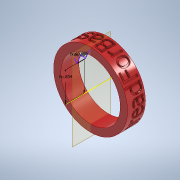
# Autodesk Inventor part: threadsForBaseV06
Saved by Autodesk Inventor 2021.1 (Build 251245010, 245A)
## iProperties
Created: 2020-08-18
Part Number: threadsForBaseV06
Material: PET Plastic
Document SubType Name: Modeling
Designer: robst
Density: 1.541 g/cm^3
Appearance: Red
Author: robst
Autodesk Inventor part; units mm, degrees
ref_plane "XZ Plane" through (0, 0, 0) normal (0, 1, 0) x (-1, 0, 0)
ref_plane "XY Plane" through (0, 0, 0) normal (0, 0, 1) x (1, 0, 0)
sketch "Sketch16" plane through (0, 0, 0) normal (0, 0, 1) x (1, 0, 0)
  circle A0 centre (0, 0) radius 21.1938
  circle A1 centre (0, 0) radius 26.3436
  dimension "d67" = 42.3875
  dimension "d68" = 52.6872
  constraints: 2 centre point, 2 coincident
  measures "d67" diameter of A0
  measures "d68" diameter of A1
extrude "Extrusion8" add sketch "Sketch16" against normal blind 12.7
ref_plane "Work Plane6" through (26.3436, 0, 0) normal (1, 0, 0) x (0, 1, 0)
sketch "Sketch18" plane through (26.3436, 0, 0) normal (1, 0, 0) x (0, 1, 0)
  line L0 (-26.3436, 0) -> (-26.3436, -12.7) projected
  line L1 (26.3436, 0) -> (26.3436, -12.7) projected
  line L2 (-26.3436, -6.35) -> (26.3436, -6.35) construction
  spline S0 degree 2 poles (-23.1079, -11.5782) (-24.1535, -11.5782) (-25.3309, -10.3844) (-25.3309, -9.0917) knots 0 0 0 1 2 2 2
  line L3 (-25.3309, -9.0917) -> (-25.3309, -4.868)
  line L4 (-25.3309, -4.868) -> (-26.1954, -4.868)
  line L5 (-26.1954, -4.868) -> (-26.1954, -3.8059)
  line L6 (-26.1954, -3.8059) -> (-25.3309, -3.8059)
  line L7 (-25.3309, -3.8059) -> (-25.3309, -1.6158)
  line L8 (-25.3309, -1.6158) -> (-24.0465, -1.6158)
  line L9 (-24.0465, -1.6158) -> (-24.0465, -3.8059)
  line L10 (-24.0465, -3.8059) -> (-21.6835, -3.8059)
  line L11 (-21.6835, -3.8059) -> (-21.6835, -4.868)
  line L12 (-21.6835, -4.868) -> (-24.0465, -4.868)
  line L13 (-24.0465, -4.868) -> (-24.0465, -8.4989)
  spline S1 degree 2 poles (-24.0465, -8.4989) (-24.0465, -9.0753) (-24.0053, -9.7092) (-23.8654, -9.9809) knots 0 0 0 1 2 2 2
  spline S2 degree 2 poles (-23.8654, -9.9809) (-23.7501, -10.2197) (-23.2314, -10.4585) (-22.7868, -10.4585) knots 0 0 0 1 2 2 2
  spline S3 degree 2 poles (-22.7868, -10.4585) (-22.4739, -10.4585) (-21.8893, -10.2691) (-21.7576, -10.2115) knots 0 0 0 1 2 2 2
  line L14 (-21.7576, -10.2115) -> (-21.6835, -10.2115)
  line L15 (-21.6835, -10.2115) -> (-21.6835, -11.3641)
  spline S4 degree 2 poles (-21.6835, -11.3641) (-22.0458, -11.4629) (-22.7868, -11.5782) (-23.1079, -11.5782) knots 0 0 0 1 2 2 2
  line L16 (-14.751, -11.43) -> (-16.0354, -11.43)
  line L17 (-16.0354, -11.43) -> (-16.0354, -7.0828)
  spline S5 degree 2 poles (-16.0354, -7.0828) (-16.0354, -6.5558) (-16.1342, -5.6502) (-16.2824, -5.3785) knots 0 0 0 1 2 2 2
  spline S6 degree 2 poles (-16.2824, -5.3785) (-16.4388, -5.0903) (-16.9987, -4.8104) (-17.4763, -4.8104) knots 0 0 0 1 2 2 2
  spline S7 degree 2 poles (-17.4763, -4.8104) (-17.9538, -4.8104) (-18.9665, -5.3208) (-19.4523, -5.7325) knots 0 0 0 1 2 2 2
  line L18 (-19.4523, -5.7325) -> (-19.4523, -11.43)
  line L19 (-19.4523, -11.43) -> (-20.7367, -11.43)
  line L20 (-20.7367, -11.43) -> (-20.7367, -0.8172)
  line L21 (-20.7367, -0.8172) -> (-19.4523, -0.8172)
  line L22 (-19.4523, -0.8172) -> (-19.4523, -4.6539)
  spline S8 degree 2 poles (-19.4523, -4.6539) (-18.8759, -4.1352) (-17.7644, -3.5918) (-17.1387, -3.5918) knots 0 0 0 1 2 2 2
  spline S9 degree 2 poles (-17.1387, -3.5918) (-16.0189, -3.5918) (-14.751, -5.0738) (-14.751, -6.4817) knots 0 0 0 1 2 2 2
  line L23 (-14.751, -6.4817) -> (-14.751, -11.43)
  line L24 (-8.9053, -5.1809) -> (-8.9712, -5.1809)
  spline S10 degree 2 poles (-8.9712, -5.1809) (-9.1194, -5.1397) (-9.4405, -5.1232) (-9.6628, -5.1232) knots 0 0 0 1 2 2 2
  spline S11 degree 2 poles (-9.6628, -5.1232) (-10.1815, -5.1232) (-11.2024, -5.5761) (-11.6635, -6.0207) knots 0 0 0 1 2 2 2
  line L25 (-11.6635, -6.0207) -> (-11.6635, -11.43)
  line L26 (-11.6635, -11.43) -> (-12.9479, -11.43)
  line L27 (-12.9479, -11.43) -> (-12.9479, -3.8059)
  line L28 (-12.9479, -3.8059) -> (-11.6635, -3.8059)
  line L29 (-11.6635, -3.8059) -> (-11.6635, -4.9421)
  spline S12 degree 2 poles (-11.6635, -4.9421) (-10.9636, -4.3164) (-9.918, -3.8059) (-9.424, -3.8059) knots 0 0 0 1 2 2 2
  spline S13 degree 2 poles (-9.424, -3.8059) (-9.2264, -3.8059) (-9.0288, -3.8223) (-8.9053, -3.8471) knots 0 0 0 1 2 2 2
  line L30 (-8.9053, -3.8471) -> (-8.9053, -5.1809)
  spline S14 degree 2 poles (-4.5992, -11.6029) (-6.427, -11.6029) (-8.436, -9.5528) (-8.436, -7.6591) knots 0 0 0 1 2 2 2
  spline S15 degree 2 poles (-8.436, -7.6591) (-8.436, -5.7984) (-6.4847, -3.5918) (-4.9121, -3.5918) knots 0 0 0 1 2 2 2
  spline S16 degree 2 poles (-4.9121, -3.5918) (-4.204, -3.5918) (-3.109, -4.0035) (-2.7056, -4.4399) knots 0 0 0 1 2 2 2
  spline S17 degree 2 poles (-2.7056, -4.4399) (-2.2939, -4.8762) (-1.8575, -6.1359) (-1.8575, -7.0498) knots 0 0 0 1 2 2 2
  line L31 (-1.8575, -7.0498) -> (-1.8575, -7.7497)
  line L32 (-1.8575, -7.7497) -> (-7.1351, -7.7497)
  spline S18 degree 2 poles (-7.1351, -7.7497) (-7.1351, -9.0753) (-5.8013, -10.4832) (-4.6157, -10.4832) knots 0 0 0 1 2 2 2
  spline S19 degree 2 poles (-4.6157, -10.4832) (-4.1958, -10.4832) (-3.3807, -10.2938) (-3.0514, -10.1456) knots 0 0 0 1 2 2 2
  spline S20 degree 2 poles (-3.0514, -10.1456) (-2.7056, -9.9809) (-2.228, -9.6928) (-2.0716, -9.561) knots 0 0 0 1 2 2 2
  line L33 (-2.0716, -9.561) -> (-1.9975, -9.561)
  line L34 (-1.9975, -9.561) -> (-1.9975, -10.9607)
  spline S21 degree 2 poles (-1.9975, -10.9607) (-2.2198, -11.0513) (-2.8949, -11.3147) (-3.1584, -11.3888) knots 0 0 0 1 2 2 2
  spline S22 degree 2 poles (-3.1584, -11.3888) (-3.5289, -11.4959) (-4.1382, -11.6029) (-4.5992, -11.6029) knots 0 0 0 1 2 2 2
  spline S23 degree 2 poles (-3.109, -6.7699) (-3.1255, -6.2512) (-3.3395, -5.4937) (-3.5454, -5.2385) knots 0 0 0 1 2 2 2
  spline S24 degree 2 poles (-3.5454, -5.2385) (-3.7677, -4.9503) (-4.4675, -4.6457) (-4.9862, -4.6457) knots 0 0 0 1 2 2 2
  spline S25 degree 2 poles (-4.9862, -4.6457) (-5.4967, -4.6457) (-6.213, -4.9503) (-6.5094, -5.2467) knots 0 0 0 1 2 2 2
  spline S26 degree 2 poles (-6.5094, -5.2467) (-6.7975, -5.5514) (-7.094, -6.2841) (-7.1351, -6.7699) knots 0 0 0 1 2 2 2
  line L35 (-7.1351, -6.7699) -> (-3.109, -6.7699)
  spline S27 degree 2 poles (3.6918, -10.6231) (3.5354, -10.7384) (3.0084, -11.1501) (2.7614, -11.2736) knots 0 0 0 1 2 2 2
  spline S28 degree 2 poles (2.7614, -11.2736) (2.4238, -11.4547) (1.7899, -11.6441) (1.2135, -11.6441) knots 0 0 0 1 2 2 2
  spline S29 degree 2 poles (1.2135, -11.6441) (0.7442, -11.6441) (-0.1038, -11.29) (-0.4249, -10.9689) knots 0 0 0 1 2 2 2
  spline S30 degree 2 poles (-0.4249, -10.9689) (-0.7295, -10.6561) (-1.1, -9.7339) (-1.1, -9.2235) knots 0 0 0 1 2 2 2
  spline S31 degree 2 poles (-1.1, -9.2235) (-1.1, -8.433) (-0.4331, -7.3133) (0.2914, -6.9922) knots 0 0 0 1 2 2 2
  spline S32 degree 2 poles (0.2914, -6.9922) (0.9336, -6.6958) (2.6791, -6.4735) (3.6918, -6.4159) knots 0 0 0 1 2 2 2
  line L36 (3.6918, -6.4159) -> (3.6918, -6.1689)
  spline S33 degree 2 poles (3.6918, -6.1689) (3.6918, -5.7243) (3.4201, -5.1726) (3.1731, -5.0162) knots 0 0 0 1 2 2 2
  spline S34 degree 2 poles (3.1731, -5.0162) (2.9261, -4.8598) (2.218, -4.761) (1.8393, -4.761) knots 0 0 0 1 2 2 2
  spline S35 degree 2 poles (1.8393, -4.761) (1.3947, -4.761) (0.1926, -5.0244) (-0.4084, -5.2797) knots 0 0 0 1 2 2 2
  line L37 (-0.4084, -5.2797) -> (-0.4825, -5.2797)
  line L38 (-0.4825, -5.2797) -> (-0.4825, -3.9706)
  spline S36 degree 2 poles (-0.4825, -3.9706) (-0.1285, -3.8718) (1.1971, -3.6247) (1.8475, -3.6247) knots 0 0 0 1 2 2 2
  spline S37 degree 2 poles (1.8475, -3.6247) (2.6379, -3.6247) (3.7165, -3.8718) (4.1446, -4.1929) knots 0 0 0 1 2 2 2
  spline S38 degree 2 poles (4.1446, -4.1929) (4.5645, -4.5057) (4.9762, -5.502) (4.9762, -6.2183) knots 0 0 0 1 2 2 2
  line L39 (4.9762, -6.2183) -> (4.9762, -11.43)
  line L40 (4.9762, -11.43) -> (3.6918, -11.43)
  line L41 (3.6918, -11.43) -> (3.6918, -10.6231)
  line L42 (3.6918, -9.5528) -> (3.6918, -7.4368)
  spline S39 degree 2 poles (3.6918, -7.4368) (3.2307, -7.478) (1.8393, -7.6179) (1.4029, -7.7497) knots 0 0 0 1 2 2 2
  spline S40 degree 2 poles (1.4029, -7.7497) (0.8924, -7.9061) (0.2255, -8.5565) (0.2255, -9.1329) knots 0 0 0 1 2 2 2
  spline S41 degree 2 poles (0.2255, -9.1329) (0.2255, -9.7916) (0.9665, -10.4585) (1.6746, -10.4585) knots 0 0 0 1 2 2 2
  spline S42 degree 2 poles (1.6746, -10.4585) (2.2756, -10.4585) (3.2637, -9.9398) (3.6918, -9.5528) knots 0 0 0 1 2 2 2
  line L43 (12.6415, -11.43) -> (11.3571, -11.43)
  line L44 (11.3571, -11.43) -> (11.3571, -10.6561)
  spline S43 degree 2 poles (11.3571, -10.6561) (11.0607, -10.9031) (10.6243, -11.2324) (10.3279, -11.3724) knots 0 0 0 1 2 2 2
  spline S44 degree 2 poles (10.3279, -11.3724) (10.0562, -11.5041) (9.4716, -11.6441) (9.0847, -11.6441) knots 0 0 0 1 2 2 2
  spline S45 degree 2 poles (9.0847, -11.6441) (8.4589, -11.6441) (7.405, -11.1254) (7.0345, -10.6231) knots 0 0 0 1 2 2 2
  spline S46 degree 2 poles (7.0345, -10.6231) (6.664, -10.1209) (6.2524, -8.6389) (6.2524, -7.6756) knots 0 0 0 1 2 2 2
  spline S47 degree 2 poles (6.2524, -7.6756) (6.2524, -6.6711) (6.7711, -5.2056) (7.2239, -4.6539) knots 0 0 0 1 2 2 2
  spline S48 degree 2 poles (7.2239, -4.6539) (7.6438, -4.1599) (8.8212, -3.5918) (9.4716, -3.5918) knots 0 0 0 1 2 2 2
  spline S49 degree 2 poles (9.4716, -3.5918) (10.0397, -3.5918) (10.8878, -3.8471) (11.3571, -4.1105) knots 0 0 0 1 2 2 2
  line L45 (11.3571, -4.1105) -> (11.3571, -0.8172)
  line L46 (11.3571, -0.8172) -> (12.6415, -0.8172)
  line L47 (12.6415, -0.8172) -> (12.6415, -11.43)
  line L48 (11.3571, -9.5775) -> (11.3571, -5.1726)
  spline S50 degree 2 poles (11.3571, -5.1726) (10.8795, -4.9421) (10.1221, -4.7692) (9.6857, -4.7692) knots 0 0 0 1 2 2 2
  spline S51 degree 2 poles (9.6857, -4.7692) (8.6977, -4.7692) (7.5779, -6.2512) (7.5779, -7.6509) knots 0 0 0 1 2 2 2
  spline S52 degree 2 poles (7.5779, -7.6509) (7.5779, -9.0012) (8.4342, -10.4255) (9.3811, -10.4255) knots 0 0 0 1 2 2 2
  spline S53 degree 2 poles (9.3811, -10.4255) (9.8833, -10.4255) (10.9042, -9.9645) (11.3571, -9.5775) knots 0 0 0 1 2 2 2
  line L49 (20.6773, -2.4721) -> (15.9513, -2.4721)
  line L50 (15.9513, -2.4721) -> (15.9513, -5.3373)
  line L51 (15.9513, -5.3373) -> (20.4797, -5.3373)
  line L52 (20.4797, -5.3373) -> (20.4797, -6.5394)
  line L53 (20.4797, -6.5394) -> (15.9513, -6.5394)
  line L54 (15.9513, -6.5394) -> (15.9513, -11.43)
  line L55 (15.9513, -11.43) -> (14.601, -11.43)
  line L56 (14.601, -11.43) -> (14.601, -1.27)
  line L57 (14.601, -1.27) -> (20.6773, -1.27)
  line L58 (20.6773, -1.27) -> (20.6773, -2.4721)
  spline S54 degree 2 poles (28.0544, -7.6179) (28.0544, -9.5446) (26.2019, -11.6441) (24.654, -11.6441) knots 0 0 0 1 2 2 2
  spline S55 degree 2 poles (24.654, -11.6441) (23.0649, -11.6441) (21.2454, -9.4787) (21.2454, -7.6179) knots 0 0 0 1 2 2 2
  spline S56 degree 2 poles (21.2454, -7.6179) (21.2454, -5.7078) (23.1226, -3.5918) (24.654, -3.5918) knots 0 0 0 1 2 2 2
  spline S57 degree 2 poles (24.654, -3.5918) (26.2019, -3.5918) (28.0544, -5.6996) (28.0544, -7.6179) knots 0 0 0 1 2 2 2
  spline S58 degree 2 poles (26.7288, -7.6179) (26.7288, -6.1359) (25.6502, -4.6951) (24.654, -4.6951) knots 0 0 0 1 2 2 2
  spline S59 degree 2 poles (24.654, -4.6951) (23.6578, -4.6951) (22.5709, -6.1359) (22.5709, -7.6179) knots 0 0 0 1 2 2 2
  spline S60 degree 2 poles (22.5709, -7.6179) (22.5709, -9.0588) (23.6578, -10.5408) (24.654, -10.5408) knots 0 0 0 1 2 2 2
  spline S61 degree 2 poles (24.654, -10.5408) (25.642, -10.5408) (26.7288, -9.0835) (26.7288, -7.6179) knots 0 0 0 1 2 2 2
  line L59 (33.4143, -5.1809) -> (33.3484, -5.1809)
  spline S62 degree 2 poles (33.3484, -5.1809) (33.2002, -5.1397) (32.8791, -5.1232) (32.6568, -5.1232) knots 0 0 0 1 2 2 2
  spline S63 degree 2 poles (32.6568, -5.1232) (32.1381, -5.1232) (31.1172, -5.5761) (30.6561, -6.0207) knots 0 0 0 1 2 2 2
  line L60 (30.6561, -6.0207) -> (30.6561, -11.43)
  line L61 (30.6561, -11.43) -> (29.3717, -11.43)
  line L62 (29.3717, -11.43) -> (29.3717, -3.8059)
  line L63 (29.3717, -3.8059) -> (30.6561, -3.8059)
  line L64 (30.6561, -3.8059) -> (30.6561, -4.9421)
  spline S64 degree 2 poles (30.6561, -4.9421) (31.356, -4.3164) (32.4016, -3.8059) (32.8956, -3.8059) knots 0 0 0 1 2 2 2
  spline S65 degree 2 poles (32.8956, -3.8059) (33.0932, -3.8059) (33.2908, -3.8223) (33.4143, -3.8471) knots 0 0 0 1 2 2 2
  line L65 (33.4143, -3.8471) -> (33.4143, -5.1809)
  spline S66 degree 2 poles (41.4007, -8.3095) (41.4007, -9.067) (40.8244, -10.2279) (40.3468, -10.6067) knots 0 0 0 1 2 2 2
  spline S67 degree 2 poles (40.3468, -10.6067) (39.7705, -11.0513) (38.4614, -11.43) (37.424, -11.43) knots 0 0 0 1 2 2 2
  line L66 (37.424, -11.43) -> (34.5094, -11.43)
  line L67 (34.5094, -11.43) -> (34.5094, -1.27)
  line L68 (34.5094, -1.27) -> (37.2017, -1.27)
  spline S68 degree 2 poles (37.2017, -1.27) (38.2885, -1.27) (39.3753, -1.41) (39.8693, -1.6817) knots 0 0 0 1 2 2 2
  spline S69 degree 2 poles (39.8693, -1.6817) (40.4209, -1.9698) (40.9232, -2.9167) (40.9232, -3.5589) knots 0 0 0 1 2 2 2
  spline S70 degree 2 poles (40.9232, -3.5589) (40.9232, -4.2752) (40.1657, -5.4114) (39.4988, -5.7325) knots 0 0 0 1 2 2 2
  line L69 (39.4988, -5.7325) -> (39.4988, -5.7819)
  spline S71 degree 2 poles (39.4988, -5.7819) (40.4045, -6.0289) (41.4007, -7.338) (41.4007, -8.3095) knots 0 0 0 1 2 2 2
  spline S72 degree 2 poles (39.9928, -8.3672) (39.9928, -7.7908) (39.6635, -7.0498) (39.1695, -6.7864) knots 0 0 0 1 2 2 2
  spline S73 degree 2 poles (39.1695, -6.7864) (38.8484, -6.6217) (38.0909, -6.5229) (37.391, -6.5229) knots 0 0 0 1 2 2 2
  line L70 (37.391, -6.5229) -> (35.8596, -6.5229)
  line L71 (35.8596, -6.5229) -> (35.8596, -10.2773)
  line L72 (35.8596, -10.2773) -> (36.9547, -10.2773)
  spline S74 degree 2 poles (36.9547, -10.2773) (37.8439, -10.2773) (38.8648, -10.1127) (39.26, -9.8492) knots 0 0 0 1 2 2 2
  spline S75 degree 2 poles (39.26, -9.8492) (39.6388, -9.5775) (39.9928, -8.9024) (39.9928, -8.3672) knots 0 0 0 1 2 2 2
  spline S76 degree 2 poles (39.5153, -3.7482) (39.5153, -3.386) (39.2683, -2.8426) (38.9966, -2.6861) knots 0 0 0 1 2 2 2
  spline S77 degree 2 poles (38.9966, -2.6861) (38.6672, -2.505) (37.8686, -2.4227) (37.1523, -2.4227) knots 0 0 0 1 2 2 2
  line L73 (37.1523, -2.4227) -> (35.8596, -2.4227)
  line L74 (35.8596, -2.4227) -> (35.8596, -5.3949)
  line L75 (35.8596, -5.3949) -> (37.391, -5.3949)
  spline S78 degree 2 poles (37.391, -5.3949) (38.025, -5.3949) (38.6261, -5.2632) (38.9472, -5.0574) knots 0 0 0 1 2 2 2
  spline S79 degree 2 poles (38.9472, -5.0574) (39.26, -4.8598) (39.5153, -4.2258) (39.5153, -3.7482) knots 0 0 0 1 2 2 2
  spline S80 degree 2 poles (46.8924, -10.6231) (46.7359, -10.7384) (46.209, -11.1501) (45.962, -11.2736) knots 0 0 0 1 2 2 2
  spline S81 degree 2 poles (45.962, -11.2736) (45.6244, -11.4547) (44.9905, -11.6441) (44.4141, -11.6441) knots 0 0 0 1 2 2 2
  spline S82 degree 2 poles (44.4141, -11.6441) (43.9448, -11.6441) (43.0968, -11.29) (42.7757, -10.9689) knots 0 0 0 1 2 2 2
  spline S83 degree 2 poles (42.7757, -10.9689) (42.471, -10.6561) (42.1005, -9.7339) (42.1005, -9.2235) knots 0 0 0 1 2 2 2
  spline S84 degree 2 poles (42.1005, -9.2235) (42.1005, -8.433) (42.7674, -7.3133) (43.492, -6.9922) knots 0 0 0 1 2 2 2
  spline S85 degree 2 poles (43.492, -6.9922) (44.1342, -6.6958) (45.8797, -6.4735) (46.8924, -6.4159) knots 0 0 0 1 2 2 2
  line L76 (46.8924, -6.4159) -> (46.8924, -6.1689)
  spline S86 degree 2 poles (46.8924, -6.1689) (46.8924, -5.7243) (46.6207, -5.1726) (46.3737, -5.0162) knots 0 0 0 1 2 2 2
  spline S87 degree 2 poles (46.3737, -5.0162) (46.1267, -4.8598) (45.4186, -4.761) (45.0399, -4.761) knots 0 0 0 1 2 2 2
  spline S88 degree 2 poles (45.0399, -4.761) (44.5953, -4.761) (43.3932, -5.0244) (42.7921, -5.2797) knots 0 0 0 1 2 2 2
  line L77 (42.7921, -5.2797) -> (42.718, -5.2797)
  line L78 (42.718, -5.2797) -> (42.718, -3.9706)
  spline S89 degree 2 poles (42.718, -3.9706) (43.0721, -3.8718) (44.3977, -3.6247) (45.0481, -3.6247) knots 0 0 0 1 2 2 2
  spline S90 degree 2 poles (45.0481, -3.6247) (45.8385, -3.6247) (46.9171, -3.8718) (47.3452, -4.1929) knots 0 0 0 1 2 2 2
  spline S91 degree 2 poles (47.3452, -4.1929) (47.7651, -4.5057) (48.1768, -5.502) (48.1768, -6.2183) knots 0 0 0 1 2 2 2
  line L79 (48.1768, -6.2183) -> (48.1768, -11.43)
  line L80 (48.1768, -11.43) -> (46.8924, -11.43)
  line L81 (46.8924, -11.43) -> (46.8924, -10.6231)
  line L82 (46.8924, -9.5528) -> (46.8924, -7.4368)
  spline S92 degree 2 poles (46.8924, -7.4368) (46.4313, -7.478) (45.0399, -7.6179) (44.6035, -7.7497) knots 0 0 0 1 2 2 2
  spline S93 degree 2 poles (44.6035, -7.7497) (44.093, -7.9061) (43.4261, -8.5565) (43.4261, -9.1329) knots 0 0 0 1 2 2 2
  spline S94 degree 2 poles (43.4261, -9.1329) (43.4261, -9.7916) (44.1671, -10.4585) (44.8752, -10.4585) knots 0 0 0 1 2 2 2
  spline S95 degree 2 poles (44.8752, -10.4585) (45.4762, -10.4585) (46.4642, -9.9398) (46.8924, -9.5528) knots 0 0 0 1 2 2 2
  spline S96 degree 2 poles (52.0382, -11.6111) (51.2725, -11.6111) (49.947, -11.1995) (49.5106, -10.9689) knots 0 0 0 1 2 2 2
  line L83 (49.5106, -10.9689) -> (49.5106, -9.5281)
  line L84 (49.5106, -9.5281) -> (49.5765, -9.5281)
  spline S97 degree 2 poles (49.5765, -9.5281) (49.7411, -9.6598) (50.1857, -9.9727) (50.5562, -10.1456) knots 0 0 0 1 2 2 2
  spline S98 degree 2 poles (50.5562, -10.1456) (50.8773, -10.302) (51.6677, -10.5326) (52.0876, -10.5326) knots 0 0 0 1 2 2 2
  spline S99 degree 2 poles (52.0876, -10.5326) (52.3923, -10.5326) (53.0921, -10.3926) (53.2568, -10.2773) knots 0 0 0 1 2 2 2
  spline S100 degree 2 poles (53.2568, -10.2773) (53.4955, -10.1209) (53.7096, -9.7669) (53.7096, -9.4046) knots 0 0 0 1 2 2 2
  spline S101 degree 2 poles (53.7096, -9.4046) (53.7096, -8.9518) (53.2156, -8.4824) (52.5816, -8.326) knots 0 0 0 1 2 2 2
  spline S102 degree 2 poles (52.5816, -8.326) (52.3346, -8.2684) (51.5442, -8.1037) (51.2067, -8.0131) knots 0 0 0 1 2 2 2
  spline S103 degree 2 poles (51.2067, -8.0131) (50.3339, -7.7579) (49.5435, -6.704) (49.5435, -5.9548) knots 0 0 0 1 2 2 2
  spline S104 degree 2 poles (49.5435, -5.9548) (49.5435, -4.9174) (51.0996, -3.6247) (52.384, -3.6247) knots 0 0 0 1 2 2 2
  spline S105 degree 2 poles (52.384, -3.6247) (53.018, -3.6247) (54.3024, -3.9376) (54.7388, -4.1764) knots 0 0 0 1 2 2 2
  line L85 (54.7388, -4.1764) -> (54.7388, -5.5514)
  line L86 (54.7388, -5.5514) -> (54.6729, -5.5514)
  spline S106 degree 2 poles (54.6729, -5.5514) (54.1789, -5.1562) (52.9768, -4.7033) (52.3593, -4.7033) knots 0 0 0 1 2 2 2
  spline S107 degree 2 poles (52.3593, -4.7033) (51.7254, -4.7033) (50.8526, -5.2385) (50.8526, -5.7737) knots 0 0 0 1 2 2 2
  spline S108 degree 2 poles (50.8526, -5.7737) (50.8526, -6.2594) (51.3713, -6.7287) (51.9477, -6.8769) knots 0 0 0 1 2 2 2
  spline S109 degree 2 poles (51.9477, -6.8769) (52.2276, -6.951) (52.9357, -7.0992) (53.3226, -7.1898) knots 0 0 0 1 2 2 2
  spline S110 degree 2 poles (53.3226, -7.1898) (54.1625, -7.4039) (55.0187, -8.3836) (55.0187, -9.2317) knots 0 0 0 1 2 2 2
  spline S111 degree 2 poles (55.0187, -9.2317) (55.0187, -9.7257) (54.6318, -10.5984) (54.253, -10.9195) knots 0 0 0 1 2 2 2
  spline S112 degree 2 poles (54.253, -10.9195) (53.8496, -11.2571) (52.8204, -11.6111) (52.0382, -11.6111) knots 0 0 0 1 2 2 2
  spline S113 degree 2 poles (59.5224, -11.6029) (57.6946, -11.6029) (55.6856, -9.5528) (55.6856, -7.6591) knots 0 0 0 1 2 2 2
  spline S114 degree 2 poles (55.6856, -7.6591) (55.6856, -5.7984) (57.6369, -3.5918) (59.2095, -3.5918) knots 0 0 0 1 2 2 2
  spline S115 degree 2 poles (59.2095, -3.5918) (59.9176, -3.5918) (61.0126, -4.0035) (61.4161, -4.4399) knots 0 0 0 1 2 2 2
  spline S116 degree 2 poles (61.4161, -4.4399) (61.8277, -4.8762) (62.2641, -6.1359) (62.2641, -7.0498) knots 0 0 0 1 2 2 2
  line L87 (62.2641, -7.0498) -> (62.2641, -7.7497)
  line L88 (62.2641, -7.7497) -> (56.9865, -7.7497)
  spline S117 degree 2 poles (56.9865, -7.7497) (56.9865, -9.0753) (58.3203, -10.4832) (59.5059, -10.4832) knots 0 0 0 1 2 2 2
  spline S118 degree 2 poles (59.5059, -10.4832) (59.9258, -10.4832) (60.7409, -10.2938) (61.0703, -10.1456) knots 0 0 0 1 2 2 2
  spline S119 degree 2 poles (61.0703, -10.1456) (61.4161, -9.9809) (61.8936, -9.6928) (62.05, -9.561) knots 0 0 0 1 2 2 2
  line L89 (62.05, -9.561) -> (62.1241, -9.561)
  line L90 (62.1241, -9.561) -> (62.1241, -10.9607)
  spline S120 degree 2 poles (62.1241, -10.9607) (61.9018, -11.0513) (61.2267, -11.3147) (60.9632, -11.3888) knots 0 0 0 1 2 2 2
  spline S121 degree 2 poles (60.9632, -11.3888) (60.5927, -11.4959) (59.9835, -11.6029) (59.5224, -11.6029) knots 0 0 0 1 2 2 2
  spline S122 degree 2 poles (61.0126, -6.7699) (60.9962, -6.2512) (60.7821, -5.4937) (60.5763, -5.2385) knots 0 0 0 1 2 2 2
  spline S123 degree 2 poles (60.5763, -5.2385) (60.354, -4.9503) (59.6541, -4.6457) (59.1354, -4.6457) knots 0 0 0 1 2 2 2
  spline S124 degree 2 poles (59.1354, -4.6457) (58.6249, -4.6457) (57.9086, -4.9503) (57.6122, -5.2467) knots 0 0 0 1 2 2 2
  spline S125 degree 2 poles (57.6122, -5.2467) (57.3241, -5.5514) (57.0277, -6.2841) (56.9865, -6.7699) knots 0 0 0 1 2 2 2
  line L91 (56.9865, -6.7699) -> (61.0126, -6.7699)
  line L92 (75.3964, -1.27) -> (71.8972, -11.43)
  line L93 (71.8972, -11.43) -> (70.4399, -11.43)
  line L94 (70.4399, -11.43) -> (66.9407, -1.27)
  line L95 (66.9407, -1.27) -> (68.3897, -1.27)
  line L96 (68.3897, -1.27) -> (71.2056, -9.7092)
  line L97 (71.2056, -9.7092) -> (74.0214, -1.27)
  line L98 (74.0214, -1.27) -> (75.3964, -1.27)
  spline S126 degree 2 poles (82.5182, -6.35) (82.5182, -9.0835) (80.9292, -11.6441) (79.2743, -11.6441) knots 0 0 0 1 2 2 2
  spline S127 degree 2 poles (79.2743, -11.6441) (77.5947, -11.6441) (76.0221, -9.0341) (76.0221, -6.3582) knots 0 0 0 1 2 2 2
  spline S128 degree 2 poles (76.0221, -6.3582) (76.0221, -3.6083) (77.6111, -1.0642) (79.2743, -1.0642) knots 0 0 0 1 2 2 2
  spline S129 degree 2 poles (79.2743, -1.0642) (80.9457, -1.0642) (82.5182, -3.6988) (82.5182, -6.35) knots 0 0 0 1 2 2 2
  spline S130 degree 2 poles (80.7728, -9.4458) (80.9704, -8.9435) (81.135, -7.3956) (81.135, -6.35) knots 0 0 0 1 2 2 2
  spline S131 degree 2 poles (81.135, -6.35) (81.135, -5.3044) (80.9704, -3.7647) (80.7645, -3.246) knots 0 0 0 1 2 2 2
  spline S132 degree 2 poles (80.7645, -3.246) (80.5587, -2.7273) (79.8424, -2.1921) (79.2743, -2.1921) knots 0 0 0 1 2 2 2
  spline S133 degree 2 poles (79.2743, -2.1921) (78.7062, -2.1921) (77.9734, -2.7273) (77.7593, -3.2625) knots 0 0 0 1 2 2 2
  spline S134 degree 2 poles (77.7593, -3.2625) (77.5535, -3.7812) (77.4053, -5.362) (77.4053, -6.3582) knots 0 0 0 1 2 2 2
  spline S135 degree 2 poles (77.4053, -6.3582) (77.4053, -7.4286) (77.537, -8.8612) (77.7511, -9.4211) knots 0 0 0 1 2 2 2
  spline S136 degree 2 poles (77.7511, -9.4211) (77.9487, -9.948) (78.6815, -10.5161) (79.2743, -10.5161) knots 0 0 0 1 2 2 2
  spline S137 degree 2 poles (79.2743, -10.5161) (79.8342, -10.5161) (80.5669, -9.9809) (80.7728, -9.4458) knots 0 0 0 1 2 2 2
  spline S138 degree 2 poles (89.9777, -8.2025) (89.9777, -8.9353) (89.5084, -10.1868) (89.0802, -10.6478) knots 0 0 0 1 2 2 2
  spline S139 degree 2 poles (89.0802, -10.6478) (88.6521, -11.1089) (87.3759, -11.6441) (86.5855, -11.6441) knots 0 0 0 1 2 2 2
  spline S140 degree 2 poles (86.5855, -11.6441) (85.861, -11.6441) (84.4449, -11.323) (83.9261, -11.0677) knots 0 0 0 1 2 2 2
  line L99 (83.9261, -11.0677) -> (83.9261, -9.6269)
  line L100 (83.9261, -9.6269) -> (84.0249, -9.6269)
  spline S141 degree 2 poles (84.0249, -9.6269) (84.1814, -9.7422) (84.766, -10.0386) (85.12, -10.1703) knots 0 0 0 1 2 2 2
  spline S142 degree 2 poles (85.12, -10.1703) (85.5234, -10.3103) (86.1903, -10.4667) (86.6102, -10.4667) knots 0 0 0 1 2 2 2
  spline S143 degree 2 poles (86.6102, -10.4667) (87.0219, -10.4667) (87.7958, -10.1703) (88.0758, -9.8492) knots 0 0 0 1 2 2 2
  spline S144 degree 2 poles (88.0758, -9.8492) (88.331, -9.5446) (88.5945, -8.7377) (88.5945, -8.1943) knots 0 0 0 1 2 2 2
  spline S145 degree 2 poles (88.5945, -8.1943) (88.5945, -7.6509) (88.2981, -6.9593) (88.0181, -6.7287) knots 0 0 0 1 2 2 2
  spline S146 degree 2 poles (88.0181, -6.7287) (87.73, -6.4735) (86.8737, -6.2594) (86.355, -6.2594) knots 0 0 0 1 2 2 2
  spline S147 degree 2 poles (86.355, -6.2594) (85.7951, -6.2594) (84.6836, -6.4323) (84.3461, -6.5064) knots 0 0 0 1 2 2 2
  line L101 (84.3461, -6.5064) -> (84.3461, -1.27)
  line L102 (84.3461, -1.27) -> (89.9201, -1.27)
  line L103 (89.9201, -1.27) -> (89.9201, -2.4638)
  line L104 (89.9201, -2.4638) -> (85.6552, -2.4638)
  line L105 (85.6552, -2.4638) -> (85.6552, -5.1726)
  spline S148 degree 2 poles (85.6552, -5.1726) (85.9022, -5.1397) (86.3797, -5.115) (86.5773, -5.115) knots 0 0 0 1 2 2 2
  spline S149 degree 2 poles (86.5773, -5.115) (87.3595, -5.115) (88.438, -5.3702) (88.932, -5.749) knots 0 0 0 1 2 2 2
  spline S150 degree 2 poles (88.932, -5.749) (89.4343, -6.1277) (89.9777, -7.2804) (89.9777, -8.2025) knots 0 0 0 1 2 2 2
  point P0 (0, 0)
  constraints: 2 end point, 2 midpoint, 1 horizontal
emboss "Emboss3" sketch "Sketch18" operation cut depth 1.27 direction (-1, 0, 0) wrap yes faces at (26.0025, -4.2258, -8.4667) contours S57 S54 L1 S61 S58 | L1 S58 S59 S60 S61 S54 S55 S56 S57 | S0 L3 L4 L5 L6 L7 L8 L9 L10 L11 L12 L13 S1 S2 S3 L14 L15 S4 | L16 L17 S5 S6 S7 L18 L19 L20 L21 L22 S8 S9 L23 | L24 S10 S11 L25 L26 L27 L28 L29 S12 S13 L30 | S14 S15 S16 S17 L31 L32 S18 S19 S20 L33 L34 S21 S22 | S27 S28 S29 S30 S31 S32 L36 S33 S34 S35 L37 L38 S36 S37 S38 L39 L40 L41 | L43 L44 S43 S44 S45 S46 S47 S48 S49 L45 L46 L47 | L49 L50 L51 L52 L53 L54 L55 L56 L57 L58 | L59 S62 S63 L60 L61 L62 L63 L64 S64 S65 L65 | S66 S67 L66 L67 L68 S68 S69 S70 L69 S71 | S80 S81 S82 S83 S84 S85 L76 S86 S87 S88 L77 L78 S89 S90 S91 L79 L80 L81 | S96 L83 L84 S97 S98 S99 S100 S101 S102 S103 S104 S105 L85 L86 S106 S107 S108 S109 S110 S111 S112 | S113 S114 S115 S116 L87 L88 S117 S118 S119 L89 L90 S120 S121 | L92 L93 L94 L95 L96 L97 L98 | S126 S127 S128 S129 | S138 S139 S140 L99 L100 S141 S142 S143 S144 S145 S146 S147 L101 L102 L103 L104 L105 S148 S149 S150
sketch "Sketch25" plane through (0, 0, 0) normal (1, 0, 0) x (0, 1, 0)
  line L0 (25.6276, 11.7571) -> (21.1938, 9.9335)
  line L1 (21.1938, 9.9335) -> (24.99, 7.0055)
  line L2 (24.99, 6.8245) -> (21.1938, 3.8966)
  line L3 (21.1938, 3.8966) -> (24.99, 0.9686)
  line L4 (21.1938, 9.9335) -> (21.1938, 3.8966)
  arc A0 (24.99, 6.8245) -> (24.99, 7.0055) centre (24.9202, 6.915) ccw
  line L5 (0, -17.7453) -> (0, 17.572) projected
  point P0 (0, 0)
  dimension "d209" = 60
  dimension "d210" = 0.1143
  dimension "d211" = 21.1938
  dimension "d212" = 25.0345
  constraints: 10 end point, 3 equal length, 2 point on circle, 2 tangent, 1 centre point, 1 parallel, 1 vertical
  measures "d209" angle of L1 L0
  measures "d210" radius of A0
  measures "d211" distance between parallel lines of L4 L5
equation "\"d67\" = b1MinorDiameter"
equation "\"d68\" = outsideDiameter"
equation "\"d209\" = threadAngle"
equation "\"d210\" = b1RootRadius"
equation "\"d211\" = 0.5 * b1MinorDiameter"
equation "\"outsideDiameter\" = 52.68722"
equation "\"b1MajorDiameter\" = 44.75226"
equation "\"b1MinorDiameter\" = 42.38752"
equation "\"b1RootRadius\" = 0.1143"
equation "\"outsideRadius\" = 0.5 * outsideDiameter"
equation "\"d142\" = outsideRadius"
equation "\"threadAngle\" = 60deg"
equation "\"secondFilet\" = 0.53642"
body "Solid3"
